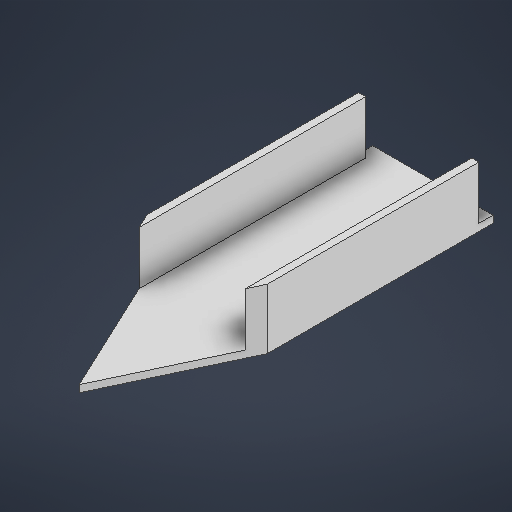
# Autodesk Inventor part: middleslide
Saved by Autodesk Inventor 2026.2 (Build 302298000, 298)
## iProperties
Created: 2026-02-23
Part Number: middleslide
Material: Generic
Document SubType Name: Sheet Metal
Designer: danda
Density: 1 g/cm^3
Sheet Metal Rule: Default_mm
Appearance: Default
Author: danda
Autodesk Inventor part; units mm, degrees
ref_plane "YZ Plane" through (0, 0, 0) normal (1, 0, 0) x (0, 1, 0)
ref_plane "XZ Plane" through (0, 0, 0) normal (0, 1, 0) x (-1, 0, 0)
ref_plane "XY Plane" through (0, 0, 0) normal (0, 0, 1) x (1, 0, 0)
sketch "Sketch1" plane through (0, 0, 0) normal (0, 0, 1) x (1, 0, 0)
  line L0 (10.7104, 9.7791) -> (40.7104, 9.7791)
  line L1 (40.7104, 9.7791) -> (40.7104, 24.7791)
  line L2 (10.7104, 9.7791) -> (10.7104, 24.7791)
  line L3 (8.7104, 24.7791) -> (8.7104, 7.7791)
  line L4 (8.7104, 7.7791) -> (42.7104, 7.7791)
  line L5 (42.7104, 7.7791) -> (42.7104, 24.7791)
  line L6 (8.7104, 24.7791) -> (10.7104, 24.7791)
  line L7 (40.7104, 24.7791) -> (42.7104, 24.7791)
  point P0 (0, 0)
  dimension "d0" = 30
  dimension "d1" = 15
  dimension "d2" = 15
  dimension "d3" = 2
  constraints: 16 end point, 3 horizontal, 2 perpendicular, 1 vertical, 2 other
  measures "d0" distance of L0.start L0.end
  measures "d1" distance of L0.end L1.end
  measures "d2" distance of L0.start L2.end
  measures "d3" distance between parallel lines of L2 L3
extrude "Extrusion1" add sketch "Sketch1" along normal blind 100
sketch "Sketch3" plane through (10.7104, 9.7791, 0) normal (0, 1, 0) x (1, 0, 0)
  line L0 (-2, -100) -> (32, -100) projected
  line L1 (-2, 0) -> (-2, -100) projected
  line L2 (15, -100) -> (37.1919, -100) construction
  line L3 (-2, -85.7353) -> (-2, -100)
  line L4 (-2, -100) -> (15, -100)
  line L5 (32, 0) -> (32, -100) projected
  line L6 (15, -100) -> (37.1919, -100) construction
  line L7 (32, -85.7353) -> (32, -100)
  line L8 (32, -100) -> (15, -100)
  line L9 (32, 0) -> (32, -100) projected
  line L10 (15, -100) -> (-2, -63.7923)
  line L11 (15, -100) -> (32, -63.7923)
  point P0 (-10.7104, 0)
  point P1 (-2, -77.7514)
  point P2 (32, -63.7923)
  dimension "d20" = 40
  dimension "d23" = 40
  constraints: 16 end point, 5 point on line, 3 collinear, 2 horizontal, 1 midpoint, 1 perpendicular
  measures "d20" distance of L2.start L10.end
  measures "d23" distance of L2.start L11.end
extrude "Extrusion5" cut sketch "Sketch3" along normal through all both and the other way through all
sketch "Sketch4" plane through (42.7104, 7.7791, 0) normal (1, 0, 0) x (0, 0, -1)
  line L0 (0, 17) -> (-68.052, 17) projected
  line L1 (0, 17) -> (-4, 17)
  line L2 (-4, 17) -> (-4, 2)
  line L3 (0, 2) -> (-68.052, 2) projected
  line L4 (0, 17) -> (0, 2) projected
  line L5 (0, 2) -> (0, 17)
  line L6 (0, 17) -> (0, 2)
  line L7 (-4, 2) -> (0, 2)
  point P0 (0, -7.7791)
  dimension "d24" = 4
  constraints: 10 end point, 2 collinear, 2 perpendicular, 2 point on line
  measures "d24" distance of L0.start L1.end
extrude "Extrusion6" cut sketch "Sketch4" against normal through all
equation "\"d23\" = d20"
equation "\"BendRadius\" = Thickness"
equation "\"BendReliefWidth\" = Thickness"
equation "\"BendReliefDepth\" = 0.5 * Thickness"
equation "\"CornerReliefSize\" = 4 * Thickness"
equation "\"MinimumRemnant\" = 2 * Thickness"
equation "\"TransitionRadius\" = BendRadius"
equation "\"JacobiRadiusSize\" = BendRadius"
equation "\"GapSize\" = Thickness"
equation "\"Thickness\" = 0.5"
body "Solid1"
